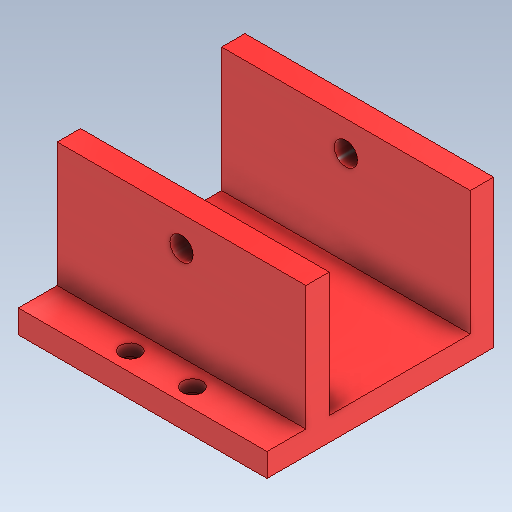
# Autodesk Inventor part: plateForPot
Saved by Autodesk Inventor 2020.2 (Build 242310000, 310)
## iProperties
Created: 2019-11-21
Part Number: plateForPot
Material: ABS Plastic
Document SubType Name: Modeling
Designer: steele
Density: 1.06 g/cm^3
Appearance: Light Red
Author: steele
Autodesk Inventor part; units mm, degrees
ref_plane "YZ Plane" through (0, 0, 0) normal (1, 0, 0) x (0, 1, 0)
ref_plane "XZ Plane" through (0, 0, 0) normal (0, 1, 0) x (-1, 0, 0)
ref_plane "XY Plane" through (0, 0, 0) normal (0, 0, 1) x (1, 0, 0)
sketch "Sketch1" plane through (0, 0, 0) normal (0, 1, 0) x (-1, 0, 0)
  line L0 (50.8, 46.2915) -> (-50.8, 46.2915)
  line L1 (-50.8, 46.2915) -> (-50.8, -46.2915)
  line L2 (-50.8, -46.2915) -> (50.8, -46.2915)
  line L3 (50.8, -46.2915) -> (50.8, 46.2915)
  line L4 (50.8, 46.2915) -> (-50.8, -46.2915) construction
  line L5 (-50.8, 46.2915) -> (50.8, -46.2915) construction
  point P0 (0, 0)
  dimension "width" = 101.6
  dimension "depth" = 92.583
  constraints: 12 end point, 2 midpoint, 2 parallel, 1 horizontal, 1 perpendicular
  measures "width" distance of L0.start L0.end
  measures "depth" distance of L1.end L0.end
extrude "Extrusion1" add sketch "Sketch1" along normal blind 9.525
sketch "Sketch2" plane through (0, 9.525, 0) normal (0, 1, 0) x (1, 0, 0)
  line L0 (-12.7, -38.6715) -> (12.7, -38.6715) construction
  line L1 (12.7, -38.6715) -> (12.7, -13.2715) construction
  line L2 (12.7, -13.2715) -> (-12.7, -13.2715) construction
  line L3 (-12.7, -13.2715) -> (-12.7, -38.6715) construction
  line L4 (-12.7, -38.6715) -> (12.7, -13.2715) construction
  line L5 (12.7, -38.6715) -> (-12.7, -13.2715) construction
  line L6 (-50.8, -46.2915) -> (50.8, -46.2915) projected
  point P0 (0, 0)
  point P1 (0, -25.9715)
  dimension "d4" = 25.4
  dimension "d5" = 25.4
  dimension "d6" = 7.62
  constraints: 12 end point, 4 coincident, 2 midpoint, 2 parallel, 1 horizontal, 1 perpendicular
  measures "d4" distance of L0.start L0.end
  measures "d5" distance of L1.end L0.end
  measures "d6" distance between parallel lines of L0 L6
hole "Hole1" at (-12.7, 9.525, 38.6715) at (12.7, 9.525, 38.6715) at (12.7, 9.525, 13.2715) at (-12.7, 9.525, 13.2715) direction (0, -1, 0) diameter 5.1054 end through all counterbore diameter 8.128 counterbore depth 4.826 clearance for "Socket Head Cap Screw" size "#10" standard "Ansi Unified Screw Threads"
sketch "Sketch3" plane through (0, 9.525, 0) normal (0, 1, 0) x (1, 0, 0)
  line L0 (-50.8, 46.2915) -> (-50.8, -46.2915) projected
  line L1 (50.8, -46.2915) -> (50.8, 46.2915) projected
  line L2 (-50.8, -30.4165) -> (50.8, -30.4165)
  line L3 (50.8, -30.4165) -> (50.8, -20.8915)
  line L4 (50.8, -20.8915) -> (-50.8, -20.8915)
  line L5 (-50.8, -20.8915) -> (-50.8, -30.4165)
  line L6 (-50.8, -46.2915) -> (50.8, -46.2915) projected
  point P0 (0, 0)
  point P1 (-50.8, -20.8915)
  point P2 (50.8, -30.4165)
  dimension "d14" = 9.525
  dimension "d16" = 25.4
  constraints: 8 end point, 2 parallel, 2 point on line, 1 horizontal, 1 perpendicular
  measures "d14" distance between parallel lines of L4 L2
  measures "d16" distance between parallel lines of L4 L6
extrude "Extrusion2" add sketch "Sketch3" along normal blind 50.8 contours L4 L1 L2 L0
sketch "Sketch5" plane through (50.8, 9.525, 20.8915) normal (0, 0, -1) x (-1, 0, 0)
  circle A0 centre (50.8, 38.5045) radius 4.7625 projected
  circle A1 centre (50.8, 38.5045) radius 4.7625
  point P0 (50.8, -9.525)
  constraints: 1 centre point, 1 coincident, 1 concentric
extrude "Extrusion4" cut sketch "Sketch5" against normal through all
sketch "Sketch6" plane through (0, 9.525, 0) normal (0, 1, 0) x (1, 0, 0)
  line L0 (50.8, 46.2915) -> (-50.8, 46.2915) projected
  line L1 (50.8, -20.8915) -> (50.8, 46.2915) projected
  line L2 (-50.8, 46.2915) -> (50.8, 46.2915)
  line L3 (50.8, 46.2915) -> (50.8, 36.7665)
  line L4 (50.8, 36.7665) -> (-50.8, 36.7665)
  line L5 (-50.8, 36.7665) -> (-50.8, 46.2915)
  point P0 (0, 0)
  dimension "d24" = 9.525
  constraints: 8 end point, 2 parallel, 1 horizontal, 1 perpendicular, 1 point on line
  measures "d24" distance of L2.end L3.end
extrude "Extrusion5" add sketch "Sketch6" along normal blind 50.8
sketch "Sketch7" plane through (-50.8, 9.525, -36.7665) normal (0, 0, 1) x (1, 0, 0)
  circle A0 centre (50.8, 38.5045) radius 4.7625 projected
  circle A1 centre (50.8, 38.5045) radius 4.7625
  point P0 (50.8, -9.525)
  constraints: 1 centre point, 1 coincident, 1 concentric
extrude "Extrusion6" cut sketch "Sketch7" against normal through all
equation "\"width\" = overallWidth"
equation "\"depth\" = overallDepth"
equation "\"overallWidth\" = 101.6"
equation "\"gapBetweeenMotorAndBasePlate\" = 0.635"
equation "\"overallDepth\" = 92.583"
body "Solid1"
